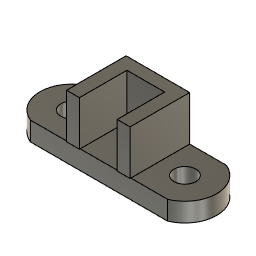
A2 (Autodesk Fusion 360 design; units mm, degrees)
Autodesk Fusion 360 part; units mm, degrees
sketch "Sketch2" plane through (0, 0, 0) normal (0, 0, 1) x (1, 0, 0)
  line L0 (57, 29.6362) -> (-57, 29.6362)
  line L1 (-57, 29.6362) -> (-57, -29.6362)
  line L2 (-57, -29.6362) -> (57, -29.6362)
  line L3 (57, -29.6362) -> (57, 29.6362)
  line L4 (57, 29.6362) -> (-57, -29.6362) construction
  line L5 (-57, 29.6362) -> (57, -29.6362) construction
  circle A0 centre (57, 0) radius 11
  circle A1 centre (-57, 0) radius 11
  line L6 (57, 29.6362) -> (69.0705, 29.6362)
  line L7 (57, -29.6362) -> (69.0705, -29.6362)
  line L8 (69.0705, 29.6362) -> (69.0705, -29.6362)
  line L9 (-57, -29.6362) -> (-69.0705, -29.6362)
  line L10 (-57, 29.6362) -> (-69.0705, 29.6362)
  line L11 (-69.0705, 29.6362) -> (-69.0705, -29.6362)
  arc A2 (-69.0705, 29.6362) -> (-69.0705, -29.6362) centre (-57, 0) ccw
  arc A3 (69.0705, -29.6362) -> (69.0705, 29.6362) centre (57, 0) ccw
  dimension "d1" = 114
  dimension "d2" = 59.2723
  dimension "d3" = 22
  dimension "d4" = 22
  dimension "d5" = 64
  dimension "d6" = 64
  constraint horizontal L0
  constraint perpendicular L0 L1
  constraint parallel L0 L2
  constraint parallel L1 L3
  constraint coincident L4 origin
  constraint coincident L5 origin
  constraint midpoint L3 A0.centre
  constraint midpoint L1 A1.centre
  constraint concentric A0 A3
  constraint concentric A1 A2
  constraint perpendicular L3 L6
  constraint perpendicular L3 L7
  constraint perpendicular L1 L9
  constraint perpendicular L1 L10
  measures "d1" distance of L1.end L2.end
  measures "d2" distance of L0.end L1.end
  measures "d3" diameter of A0
  measures "d4" diameter of A1
  measures "d5" diameter of A3
  measures "d6" diameter of A2
extrude "Extrude1" add sketch "Sketch2" along normal blind 19 contours L0 L1 L2 L3 A0 A1 | L3 A0 L6 L7 L8 | L1 A1 L9 L10 L11 | L8 A3 | L11 A2
sketch "Sketch3" plane through (0, 0, 19) normal (0, 0, 1) x (-1, 0, 0)
  circle A0 centre (57, 0) radius 11
  circle A1 centre (-57, 0) radius 11
  line L0 (69.0705, 29.6362) -> (-69.0705, 29.6362)
  arc A2 (-69.0705, 29.6362) -> (-69.0705, -29.6362) centre (-57, 0) ccw
  line L1 (-69.0705, -29.6362) -> (69.0705, -29.6362)
  arc A3 (69.0705, -29.6362) -> (69.0705, 29.6362) centre (57, 0) ccw
  line L2 (32, -29.6362) -> (32, 29.6362) construction
  line L3 (-32, -29.6362) -> (-32, 29.6362) construction
  dimension "d9" = 64
  dimension "d10" = 25
  constraint coincident L1 L2.start
  constraint perpendicular L1 L2
  constraint coincident L0 L2.end
  constraint coincident L1 L3.start
  constraint perpendicular L1 L3
  constraint coincident L0 L3.end
  measures "d9" distance of L2 L3
  measures "d10" distance of A0.centre L2
sketch "Sketch4" plane through (0, 29.6362, 0) normal (0, 1, 0) x (-1, 0, 0)
  line L0 (-69.0705, 0) -> (69.0705, 0)
  line L1 (69.0705, 0) -> (69.0705, 19)
  line L2 (69.0705, 19) -> (-69.0705, 19)
  line L3 (-69.0705, 19) -> (-69.0705, 0)
  line L4 (-32.0857, 19) -> (31.9143, 19)
  line L5 (31.9143, 19) -> (31.9143, 64)
  line L6 (31.9143, 64) -> (-32.0857, 64)
  line L7 (-32.0857, 64) -> (-32.0857, 19)
  dimension "d11" = 64
  dimension "d12" = 45
  constraint horizontal L4
  constraint vertical L5
  constraint horizontal L6
  constraint vertical L7
  constraint coincident L2 L4.start
  measures "d11" distance of L4.start L4.end
  measures "d12" distance of L4.start L6.end
extrude "Extrude2" add sketch "Sketch4" against normal blind 60 contours L2 L4 L5 L6 L7
sketch "Sketch5" plane through (0, 0, 64) normal (0, 0, 1) x (-1, 0, 0)
  line L0 (-32.0857, -29.6362) -> (31.9143, -29.6362)
  line L1 (31.9143, -29.6362) -> (31.9143, 30.3638)
  line L2 (31.9143, 30.3638) -> (-32.0857, 30.3638)
  line L3 (-32.0857, 30.3638) -> (-32.0857, -29.6362)
  line L4 (31.9143, -17.4462) -> (-32.0857, -17.4462)
  line L5 (18.9143, -17.4462) -> (18.9143, 30.3638)
  line L6 (-19.0857, -17.4462) -> (-19.0857, 30.3638)
  dimension "d15" = 12.19
  dimension "d16" = 38
  dimension "d17" = 13
  constraint coincident L1 L4.start
  constraint perpendicular L1 L4
  constraint coincident L3 L4.end
  constraint coincident L4 L5.start
  constraint perpendicular L4 L5
  constraint coincident L2 L5.end
  constraint coincident L4 L6.start
  constraint perpendicular L4 L6
  constraint coincident L2 L6.end
  measures "d15" distance of L0 L4
  measures "d16" distance of L5 L6
  measures "d17" distance of L1 L5
extrude "Extrude3" cut sketch "Sketch5" against normal blind 45 contours L2 L4 L5 L6
equation "d12 = 64 mm - 19 mm"
